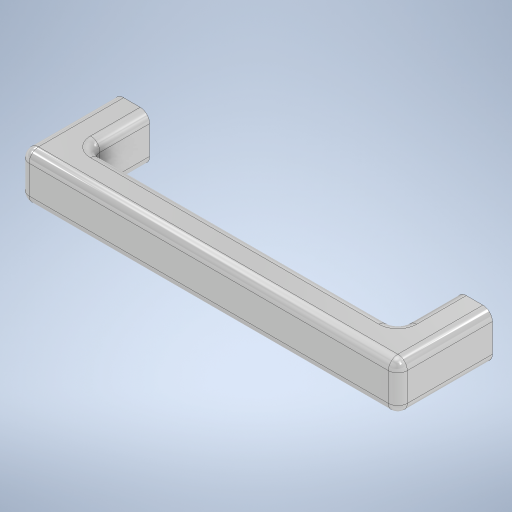
# Autodesk Inventor part: Handle
Saved by Autodesk Inventor 2024 (Build 280153000, 153)
## iProperties
Created: 2023-06-26
Part Number: Handle
Material: Generic
Document SubType Name: Modeling
Designer: 69
Density: 1 g/cm^3
Appearance: Default
Author: 69
Autodesk Inventor part; units mm, degrees
ref_plane "YZ Plane" through (0, 0, 0) normal (1, 0, 0) x (0, 1, 0)
ref_plane "XZ Plane" through (0, 0, 0) normal (0, 1, 0) x (-1, 0, 0)
ref_plane "XY Plane" through (0, 0, 0) normal (0, 0, 1) x (1, 0, 0)
sketch "Sketch4" plane through (0, 0, 0) normal (0, 0, 1) x (1, 0, 0)
  line L0 (-80, 10) -> (80, 10)
  line L1 (80, 10) -> (80, -10)
  line L2 (80, -10) -> (-80, -10)
  line L3 (-80, -10) -> (-80, 10)
  line L4 (-80, 10) -> (80, -10) construction
  line L5 (80, 10) -> (-80, -10) construction
  point P0 (0, 0)
  dimension "d33" = 160
  dimension "d34" = 20
  constraints: 12 end point, 2 midpoint, 2 parallel, 1 horizontal, 1 perpendicular
  measures "d33" distance of L1.end L2.end
  measures "d34" distance of L0.end L1.end
extrude "Extrusion1" add sketch "Sketch4" along normal blind 40
sketch "Sketch5" plane through (-80, 10, 0) normal (0, 1, 0) x (1, 0, 0)
  line L0 (0, 0) -> (160, 0) projected
  line L1 (15, 0) -> (145, 0)
  line L2 (145, 0) -> (145, -25)
  line L3 (145, -25) -> (15, -25)
  line L4 (15, -25) -> (15, 0)
  line L5 (160, -40) -> (0, -40) projected
  line L6 (160, 0) -> (160, -40) projected
  line L7 (0, 0) -> (0, -40) projected
  point P0 (80, 0)
  point P1 (0, -20)
  dimension "d37" = 15
  dimension "d38" = 15
  dimension "d39" = 15
  constraints: 8 end point, 2 parallel, 1 horizontal, 1 midpoint, 1 perpendicular, 1 point on line
  measures "d37" distance between parallel lines of L5 L3
  measures "d38" distance between parallel lines of L6 L2
  measures "d39" distance from line of point (0, -20) L4
extrude "Extrusion2" cut sketch "Sketch5" against normal blind 40 contours L0 L2 L3 L4
fillet "Fillet1" radius 4 16 edges at (80, 0, 40) (0, 10, 40) (0, -10, 40) (80, 10, 20) (80, -10, 20) (0, 10, 25) (65, 10, 12.5) (0, -10, 25) (65, -10, 12.5) (65, 0, 25) (-65, -10, 12.5) (-65, 0, 25) (-65, 10, 12.5) (-80, -10, 20) (-80, 10, 20) (-80, 0, 40)
body "Solid2"
